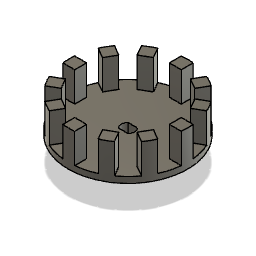
RobotWheel (Autodesk Fusion 360 design; units mm, degrees)
Autodesk Fusion 360 part; units mm, degrees
sketch "Sketch1" plane through (0, 0, 0) normal (0, 1, 0) x (1, 0, 0)
  circle A0 centre (0, 0) radius 2.805
  line L0 (-2.805, 2) -> (2.805, 2)
  line L1 (2.805, 2) -> (2.805, -2)
  line L2 (2.805, -2) -> (-2.805, -2)
  line L3 (-2.805, -2) -> (-2.805, 2)
  line L4 (0, 2) -> (0, 0) construction
  line L5 (0, 0) -> (0, -2) construction
  circle A1 centre (0, 0) radius 5
  dimension "d1" = 5.61
  dimension "d2" = 2
  dimension "d3" = 10
  constraint coincident A0.centre L4.end
  constraint horizontal L0
  constraint vertical L1
  constraint horizontal L2
  constraint vertical L3
  constraint tangent A0 L3
  constraint tangent A0 L1
  constraint midpoint L0 L4.start
  constraint midpoint L2 L5.end
  constraint equal L4 L5
  constraint concentric A0 A1
  measures "d1" diameter of A0
  measures "d2" distance of L4.start A0.centre
  measures "d3" diameter of A1
extrude "Extrude1" add sketch "Sketch1" along normal blind 10 contours A0 L1 L2 | A0 L0 L1 | A0 L0 | A0 L2 | A0 L0 L3 | A0 L2 L3 | A1
sketch "Sketch2" plane through (0, 10, 0) normal (0, 1, 0) x (-1, 0, 0)
  arc A0 (1.9667, -2) -> (1.9667, 2) centre (0, 0) ccw
  line L0 (1.9667, -2) -> (-1.9667, -2)
  arc A1 (-1.9667, 2) -> (-1.9667, -2) centre (0, 0) ccw
  line L1 (-1.9667, 2) -> (1.9667, 2)
  circle A2 centre (0, 0) radius 5
  circle A3 centre (0, 0) radius 25
  line L2 (-2.5, -24.8747) -> (-2.5, -19.8747)
  line L3 (-2.5, -19.8747) -> (2.5, -19.8747)
  line L4 (2.5, -19.8747) -> (2.5, -24.8747)
  line L5 (12.1024, -15.962) -> (14.6024, -20.2921)
  line L6 (7.7723, -18.462) -> (12.1024, -15.962)
  line L7 (10.2723, -22.7921) -> (7.7723, -18.462)
  line L8 (18.462, -7.7723) -> (22.7921, -10.2723)
  line L9 (15.962, -12.1024) -> (18.462, -7.7723)
  line L10 (20.2921, -14.6024) -> (15.962, -12.1024)
  line L11 (19.8747, 2.5) -> (24.8747, 2.5)
  line L12 (19.8747, -2.5) -> (19.8747, 2.5)
  line L13 (24.8747, -2.5) -> (19.8747, -2.5)
  line L14 (15.962, 12.1024) -> (20.2921, 14.6024)
  line L15 (18.462, 7.7723) -> (15.962, 12.1024)
  line L16 (22.7921, 10.2723) -> (18.462, 7.7723)
  line L17 (7.7723, 18.462) -> (10.2723, 22.7921)
  line L18 (12.1024, 15.962) -> (7.7723, 18.462)
  line L19 (14.6024, 20.2921) -> (12.1024, 15.962)
  line L20 (-2.5, 19.8747) -> (-2.5, 24.8747)
  line L21 (2.5, 19.8747) -> (-2.5, 19.8747)
  line L22 (2.5, 24.8747) -> (2.5, 19.8747)
  line L23 (-12.1024, 15.962) -> (-14.6024, 20.2921)
  line L24 (-7.7723, 18.462) -> (-12.1024, 15.962)
  line L25 (-10.2723, 22.7921) -> (-7.7723, 18.462)
  line L26 (-18.462, 7.7723) -> (-22.7921, 10.2723)
  line L27 (-15.962, 12.1024) -> (-18.462, 7.7723)
  line L28 (-20.2921, 14.6024) -> (-15.962, 12.1024)
  line L29 (-19.8747, -2.5) -> (-24.8747, -2.5)
  line L30 (-19.8747, 2.5) -> (-19.8747, -2.5)
  line L31 (-24.8747, 2.5) -> (-19.8747, 2.5)
  line L32 (-15.962, -12.1024) -> (-20.2921, -14.6024)
  line L33 (-18.462, -7.7723) -> (-15.962, -12.1024)
  line L34 (-22.7921, -10.2723) -> (-18.462, -7.7723)
  line L35 (-7.7723, -18.462) -> (-10.2723, -22.7921)
  line L36 (-12.1024, -15.962) -> (-7.7723, -18.462)
  line L37 (-14.6024, -20.2921) -> (-12.1024, -15.962)
  dimension "d6" = 50
  dimension "d7" = 5
  dimension "d9" = 360
  constraint concentric A0 A3
  constraint vertical L2
  constraint horizontal L3
  constraint vertical L4
  constraint coincident A3 L2.start
  constraint coincident A3 L4.end
  constraint equal L3 L4
  constraint equal L2 L4
  measures "d6" diameter of A3
  measures "d7" distance of L4.end L3.end
extrude "Extrude2" add sketch "Sketch2" along normal blind 2.5 contours A2 | A3 L2 L3 L4 L5 L6 L7 L8 L9 L10 L11 L12 L13 L14 L15 L16 L17 L18 L19 L20 L21 L22 L23 L24 L25 L26 L27 L28 L29 L30 L31 L32 L33 L34 L35 L36 L37
extrude "Extrude3" add sketch "Sketch2" along normal blind 15 contours A3 L11 L12 L13 | A3 L14 L15 L16 | A3 L8 L9 L10 | A3 L17 L18 L19 | A3 L5 L6 L7 | A3 L20 L21 L22 | A3 L2 L3 L4 | A3 L23 L24 L25 | A3 L35 L36 L37 | A3 L26 L27 L28 | A3 L32 L33 L34 | A3 L29 L30 L31
equation "d1 = ( 5.5 * 1.02 ) * 1 mm"
